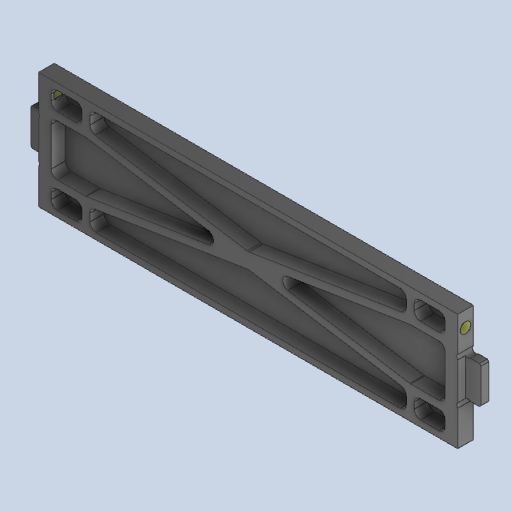
# Autodesk Inventor part: Cockpit_battery_frame
Saved by Autodesk Inventor 2022.3 (Build 263350000, 350)
## iProperties
Part Number: Cockpit_battery_frame
Material: アセタール樹脂、黒
Document SubType Name: Modeling
Designer: Masato Kubotera
Density: 1.425 g/cm^3
Appearance: 滑らか - 黒
Description: POM T5
Mass: 13.79 g
Surface Area: 149.623 cm^2
Volume: 9.6772 cm^3
Author: Masato Kubotera
Autodesk Inventor part; units mm, degrees
ref_plane "XZ Plane" through (0, 0, 0) normal (0, 1, 0) x (-1, 0, 0)
derived "Cockpit_side_frame.ipt"
sketch "スケッチ2" plane through (0, 0, 0) normal (0, 1, 0) x (-1, 0, 0)
  line L0 (-23.5, -22.5) -> (-28.5, -27.5)
  line L1 (-28.5, -27.5) -> (-28.5, -91)
  line L2 (-28.5, -91) -> (-23.5, -96)
  line L3 (-23.5, -96) -> (34.25, -96)
  line L4 (36.25, -98) -> (36.25, -128.5)
  line L5 (36.25, -128.5) -> (46.25, -138.5)
  line L6 (46.25, -138.5) -> (86.5, -138.5)
  line L7 (91.5, -133.5) -> (91.5, -20)
  line L8 (91.5, -20) -> (89, -17.5)
  line L9 (89, -17.5) -> (83.25, -17.5)
  line L10 (83.25, -17.5) -> (83.25, -21.0151)
  line L11 (81.7651, -22.5) -> (76.8599, -22.5)
  line L12 (75.375, -21.0151) -> (75.375, -17.5)
  line L13 (75.375, -17.5) -> (60.375, -17.5)
  line L14 (60.375, -17.5) -> (60.375, -21.0151)
  line L15 (58.8901, -22.5) -> (-23.5, -22.5)
  line L16 (-25.25, -25) -> (-20.25, -25) construction
  line L17 (-20.25, -25) -> (-20.25, -93.5) construction
  line L18 (-20.25, -93.5) -> (-25.25, -93.5) construction
  line L19 (-25.25, -93.5) -> (-25.25, -25) construction
  line L20 (-26, -25) -> (-25.25, -25) construction
  line L21 (-25.25, -93.5) -> (-26, -93.5) construction
  line L22 (-26, -93.5) -> (-26, -25) construction
  line L23 (-20.25, -93.5) -> (83.25, -93.5) construction
  line L24 (-20.25, -88.5) -> (83.25, -88.5) construction
  line L25 (83.25, -22.5) -> (83.25, -90) construction
  line L26 (83.25, -90) -> (88.25, -90) construction
  line L27 (88.25, -90) -> (88.25, -22.5) construction
  line L28 (83.25, -88.5) -> (83.25, -93.5) construction
  line L29 (83.25, -91) -> (88.25, -91) construction
  line L30 (88.25, -91) -> (88.25, -136) construction
  line L31 (83.25, -91) -> (83.25, -136) construction
  line L32 (83.25, -136) -> (88.25, -136) construction
  line L33 (38.75, -131) -> (38.75, -93.5) construction
  line L34 (43.75, -93.5) -> (43.75, -131) construction
  line L35 (38.75, -131) -> (43.75, -131) construction
  line L36 (41.25, -131) -> (41.25, -93.5) construction
  line L37 (43.75, -131) -> (81.25, -131) construction
  line L38 (81.25, -131) -> (81.25, -136) construction
  line L39 (81.25, -136) -> (43.75, -136) construction
  line L40 (43.75, -133.5) -> (81.25, -133.5) construction
  line L41 (85.75, -91) -> (85.75, -136) construction
  circle A0 centre (85.75, -133.5) radius 2.975
  arc A1 (83.25, -131) -> (88.25, -131) centre (85.75, -133.5) ccw construction
  line L42 (83.25, -91) -> (-20.25, -91) construction
  line L43 (41.25, -112.25) -> (43.75, -112.25) construction
  line L44 (62.5, -131) -> (62.5, -133.5) construction
  line L45 (41.2, -116.8151) -> (41.2, -107.6849)
  line L46 (43.8, -108.3) -> (43.8, -116.2)
  line L47 (43.8, -118.3) -> (41.2, -106.2) construction
  line L48 (41.2, -118.3) -> (43.8, -106.2) construction
  line L49 (58.55, -130.95) -> (66.45, -130.95)
  line L50 (67.0651, -133.55) -> (57.9349, -133.55)
  line L51 (56.45, -130.95) -> (68.55, -133.55) construction
  line L52 (68.55, -130.95) -> (56.45, -133.55) construction
  line L53 (41.25, -106.25) -> (43.75, -106.25) construction
  line L54 (41.25, -118.25) -> (43.75, -118.25) construction
  arc A2 (42.6849, -106.2) -> (41.2, -107.6849) centre (41.9425, -106.9425) ccw
  arc A3 (43.8, -108.3) -> (43.8, -106.2) centre (43.8, -107.25) ccw
  arc A4 (41.2, -116.8151) -> (42.6849, -118.3) centre (41.9425, -117.5575) ccw
  arc A5 (43.8, -118.3) -> (43.8, -116.2) centre (43.8, -117.25) ccw
  line L55 (56.5, -133.5) -> (56.5, -131) construction
  line L56 (68.5, -131) -> (68.5, -133.5) construction
  arc A6 (56.45, -132.0651) -> (57.9349, -133.55) centre (57.1925, -132.8075) ccw
  arc A7 (58.55, -130.95) -> (56.45, -130.95) centre (57.5, -130.95) ccw
  arc A8 (67.0651, -133.55) -> (68.55, -132.0651) centre (67.8075, -132.8075) ccw
  arc A9 (68.55, -130.95) -> (66.45, -130.95) centre (67.5, -130.95) ccw
  line L57 (56.45, -132.0651) -> (56.45, -130.95)
  line L58 (68.55, -130.95) -> (68.55, -132.0651)
  line L59 (42.6849, -106.2) -> (43.8, -106.2)
  line L60 (43.8, -118.3) -> (42.6849, -118.3)
  circle A10 centre (48.75, -133.5) radius 1.6
  line L61 (88.25, -22.5) -> (88.25, -17.5) construction
  line L62 (89, -17.5) -> (89, -90) construction
  line L63 (89, -90) -> (88.25, -90) construction
  line L64 (-13.5, -82.5) -> (-13.5, -61)
  arc A11 (-13.5, -82.5) -> (-11.5, -84.5) centre (-11.5, -82.5) ccw
  line L65 (45.5, -84.5) -> (-11.5, -84.5)
  arc A12 (45.5, -84.5) -> (47.5, -82.5) centre (45.5, -82.5) ccw
  line L66 (47.5, -61) -> (47.5, -82.5)
  arc A13 (47.5, -61) -> (45.5, -59) centre (45.5, -61) ccw
  line L67 (-11.5, -59) -> (45.5, -59)
  arc A14 (-11.5, -59) -> (-13.5, -61) centre (-11.5, -61) ccw
  line L68 (31.5, -88.5) -> (31.5, -91) construction
  line L69 (85.75, -22.5) -> (85.75, -90) construction
  circle A15 centre (85.75, -31.25) radius 1.6
  circle A16 centre (85.75, -31.25) radius 3
  circle A17 centre (85.75, -81.25) radius 3
  circle A18 centre (85.75, -81.25) radius 1.6
  line L70 (88.25, -22.5) -> (83.25, -22.5) construction
  arc A19 (88.25, -91) -> (83.25, -91) centre (85.75, -133.5) ccw construction
  circle A20 centre (48.75, -133.5) radius 3
  circle A21 centre (41.25, -98.5) radius 1.6
  circle A22 centre (41.25, -98.5) radius 3
  line L71 (10.55, -88.5) -> (10.55, -91) construction
  line L72 (52.45, -88.5) -> (52.45, -91) construction
  line L73 (51.0151, -91.05) -> (11.9849, -91.05)
  line L74 (10.5, -89.5651) -> (10.5, -88.45)
  line L75 (12.6, -88.45) -> (50.4, -88.45)
  line L76 (52.5, -88.45) -> (52.5, -89.5651)
  line L77 (52.5, -91.05) -> (10.5, -88.45) construction
  line L78 (10.5, -91.05) -> (52.5, -88.45) construction
  arc A23 (12.6, -88.45) -> (10.5, -88.45) centre (11.55, -88.45) ccw
  arc A24 (10.5, -89.5651) -> (11.9849, -91.05) centre (11.2425, -90.3075) ccw
  arc A25 (51.0151, -91.05) -> (52.5, -89.5651) centre (51.7575, -90.3075) ccw
  arc A26 (52.5, -88.45) -> (50.4, -88.45) centre (51.45, -88.45) ccw
  line L79 (-20.25, -31) -> (83.25, -31) construction
  line L80 (83.25, -26) -> (-20.25, -26) construction
  line L81 (-20.25, -26) -> (-20.25, -31) construction
  line L82 (-20.25, -28.5) -> (83.25, -28.5) construction
  line L83 (31.5, -31) -> (31.5, -26) construction
  line L84 (11.9849, -31) -> (51.0151, -31)
  arc A27 (10.5, -29.5151) -> (11.9849, -31) centre (11.2425, -30.2575) ccw
  arc A28 (51.0151, -31) -> (52.5, -29.5151) centre (51.7575, -30.2575) ccw
  line L85 (10.55, -31) -> (10.55, -26) construction
  line L86 (52.45, -26) -> (52.45, -31) construction
  circle A29 centre (6.5, -28.5) radius 1.6
  circle A30 centre (6.5, -28.5) radius 3
  line L87 (-26, -59.25) -> (-25.25, -59.25) construction
  line L88 (-22.75, -25) -> (-22.75, -93.5) construction
  arc A31 (58.8901, -22.5) -> (60.375, -21.0151) centre (59.6325, -21.7575) ccw
  arc A32 (75.375, -21.0151) -> (76.8599, -22.5) centre (76.1175, -21.7575) ccw
  line L89 (56.4375, -22.5) -> (56.4375, -17.5) construction
  line L90 (79.3125, -22.5) -> (79.3125, -17.5) construction
  circle A33 centre (-22.75, -31.75) radius 1.6
  circle A34 centre (-22.75, -31.75) radius 3
  circle A35 centre (-22.75, -86.75) radius 1.6
  circle A36 centre (-22.75, -86.75) radius 3
  line L91 (60.375, -22.5) -> (75.375, -22.5)
  line L92 (52.5, -17.5) -> (52.5, -22.5) construction
  circle A37 centre (85.75, -98.5) radius 1.475
  circle A38 centre (85.75, -103.5) radius 1.475
  circle A39 centre (85.75, -108.5) radius 1.475
  line L93 (59.5, -88.5) -> (78.75, -88.5)
  line L94 (80.75, -90.5) -> (80.75, -126.5)
  line L95 (78.75, -128.5) -> (48.25, -128.5)
  line L96 (46.25, -126.5) -> (46.25, -110)
  arc A40 (46.25, -126.5) -> (48.25, -128.5) centre (48.25, -126.5) ccw
  arc A41 (78.75, -128.5) -> (80.75, -126.5) centre (78.75, -126.5) ccw
  arc A42 (80.75, -90.5) -> (78.75, -88.5) centre (78.75, -90.5) ccw
  arc A43 (36.25, -98) -> (34.25, -96) centre (34.25, -98) ccw
  circle A44 centre (-13.5, -55) radius 1.75
  circle A45 centre (-13.5, -55) radius 2
  line L97 (23.9, -43.85) -> (10.1, -43.85) construction
  line L98 (10.1, -43.85) -> (10.1, -34.65) construction
  line L99 (10.1, -34.65) -> (23.9, -34.65) construction
  line L100 (23.9, -34.65) -> (23.9, -43.85) construction
  line L101 (23.9, -43.85) -> (10.1, -34.65) construction
  line L102 (10.1, -43.85) -> (23.9, -34.65) construction
  line L103 (9.45, -33.95) -> (24.55, -33.95) construction
  line L104 (24.55, -33.95) -> (24.55, -44.55) construction
  line L105 (24.55, -44.55) -> (9.45, -44.55) construction
  line L106 (9.45, -44.55) -> (9.45, -33.95) construction
  line L107 (9.45, -33.95) -> (24.55, -44.55) construction
  line L108 (24.55, -33.95) -> (9.45, -44.55) construction
  line L109 (10.8849, -33.9) -> (23.1151, -33.9)
  line L110 (24.6, -35.3849) -> (24.6, -43.1151)
  line L111 (24.6, -44.6) -> (9.4, -33.9) construction
  line L112 (9.4, -44.6) -> (24.6, -33.9) construction
  line L113 (23.95, -43.9) -> (10.05, -34.6) construction
  line L114 (10.05, -43.9) -> (23.95, -34.6) construction
  arc A46 (10.8849, -33.9) -> (9.4, -35.3849) centre (10.1425, -34.6425) ccw
  arc A47 (11.5349, -34.6) -> (10.05, -36.0849) centre (10.7925, -35.3425) ccw
  line L115 (9.4, -39.25) -> (24.6, -39.25) construction
  line L116 (17, -33.9) -> (17, -44.6) construction
  arc A48 (24.6, -35.3849) -> (23.1151, -33.9) centre (23.8575, -34.6425) ccw
  arc A49 (23.95, -36.0849) -> (22.4651, -34.6) centre (23.2075, -35.3425) ccw
  arc A50 (10.05, -42.4151) -> (11.5349, -43.9) centre (10.7925, -43.1575) ccw
  arc A51 (9.4, -43.1151) -> (10.8849, -44.6) centre (10.1425, -43.8575) ccw
  arc A52 (22.4651, -43.9) -> (23.95, -42.4151) centre (23.2075, -43.1575) ccw
  arc A53 (23.1151, -44.6) -> (24.6, -43.1151) centre (23.8575, -43.8575) ccw
  line L117 (11.5349, -34.6) -> (22.4651, -34.6)
  line L118 (23.95, -36.0849) -> (23.95, -42.4151)
  line L119 (9.4, -43.1151) -> (9.4, -35.3849)
  line L120 (10.05, -42.4151) -> (10.05, -36.0849)
  line L121 (22.4651, -43.9) -> (11.5349, -43.9)
  line L122 (23.1151, -44.6) -> (10.8849, -44.6)
  line L123 (-13.5, -71.75) -> (47.5, -71.75) construction
  line L124 (85.75, -56.25) -> (88.25, -56.25) construction
  line L125 (85.7, -69.2) -> (85.7, -43.3)
  line L126 (88.3049, -71.3569) -> (85.7, -41.2) construction
  line L127 (85.7, -71.3) -> (88.3, -41.2) construction
  arc A54 (85.7, -41.2) -> (85.7, -43.3) centre (85.7, -42.25) ccw
  arc A55 (88.3, -42.6849) -> (86.8151, -41.2) centre (87.5575, -41.9425) ccw
  arc A56 (85.7, -69.2) -> (85.7, -71.3) centre (85.7, -70.25) ccw
  arc A57 (86.8151, -71.3) -> (88.3, -69.8151) centre (87.5575, -70.5575) ccw
  line L128 (85.75, -41.25) -> (88.25, -41.25) construction
  line L129 (85.75, -71.25) -> (88.25, -71.25) construction
  line L130 (88.3, -42.6849) -> (88.3, -69.8151)
  line L131 (88.3, -66.8652) -> (88.3, -69.8151)
  line L132 (86.8151, -71.3) -> (85.7, -71.3)
  line L133 (85.7, -41.2) -> (86.8151, -41.2)
  line L134 (86.5, -138.5) -> (91.5, -133.5)
  arc A58 (81.7651, -22.5) -> (83.25, -21.0151) centre (82.5075, -21.7575) ccw
  circle A59 centre (85.75, -93.5) radius 2
  circle A60 centre (85.75, -93.5) radius 4 construction
  arc A61 (-13.5, -49) -> (-11.5, -51) centre (-11.5, -49) ccw construction
  line L135 (45.5, -51) -> (-11.5, -51) construction
  arc A62 (45.5, -51) -> (47.5, -49) centre (45.5, -49) ccw construction
  line L136 (10.5, -29.5151) -> (10.5, -22.5)
  line L137 (52.5, -29.5151) -> (52.5, -22.5)
  line L138 (67.875, -17.5) -> (67.875, -22.5) construction
  line L139 (52.5, -17.5) -> (83.25, -17.5) construction
  line L140 (43.75, -131) -> (43.75, -136) construction
  line L141 (57.5, -22.5) -> (57.5, -103) construction
  line L142 (57.5, -103) -> (52.5, -108) construction
  line L143 (-23.5, -108) -> (52.5, -108) construction
  line L144 (57.5, -90.5) -> (57.5, -103)
  line L145 (57.5, -103) -> (52.5, -108)
  line L146 (52.5, -108) -> (48.25, -108)
  arc A63 (59.5, -88.5) -> (57.5, -90.5) centre (59.5, -90.5) ccw
  arc A64 (48.25, -108) -> (46.25, -110) centre (48.25, -110) ccw
  circle A65 centre (56.5, -28.5) radius 3
  circle A66 centre (56.5, -28.5) radius 1.6
  line L147 (-13.5, -49) -> (-13.5, -29.5)
  point P0 (0, 0)
  point P1 (-25.7227, -96)
  point P2 (-23.5, -22.5)
  point P3 (42.5, -112.25)
  point P4 (62.5, -132.25)
  point P5 (31.5, -89.75)
  point P6 (31.5, -28.5)
  point P7 (52.5, -22)
  point P8 (46.25, -108)
  point P9 (57.5, -88.5)
  point P10 (17, -39.25)
  point P11 (17, -39.25)
  point P12 (87, -56.25)
  point P13 (17, -51)
  point P14 (10.5, -31)
  point P15 (-13.5, -39.25)
  dimension "d1" = 43.75
  dimension "d2" = 5
  dimension "d3" = 2.5
  measures "d1" distance from line of point (0, 0) L34
  measures "d2" distance of L34.end L33.start
  measures "d3" distance of L54.start L54.end
ref_plane "作業平面1" through (-43.75, 0, 0) normal (1, 0, 0) x (0, 1, 0)
sketch "スケッチ3" plane through (-43.75, 0, 0) normal (1, 0, 0) x (0, 1, 0)
  line L0 (-135, -93.5) -> (0, -93.5)
  line L1 (0, -131) -> (-135, -131)
  line L2 (1.4849, -106.25) -> (5, -106.25)
  line L3 (5, -106.25) -> (5, -118.25)
  arc A0 (0, -104.7651) -> (1.4849, -106.25) centre (0.7425, -105.5075) ccw
  line L4 (0, -93.5) -> (0, -104.7651)
  line L5 (-134.9908, -112.25) -> (0, -112.25) construction
  line L6 (1.4849, -118.25) -> (5, -118.25)
  arc A1 (1.4849, -118.25) -> (0, -119.7349) centre (0.7425, -118.9925) ccw
  line L7 (0, -131) -> (0, -119.7349)
  line L8 (0, -106.25) -> (0, -118.25)
  line L9 (0, -119.7349) -> (0, -131)
  line L10 (-67.5, -93.5) -> (-67.5, -131) construction
  line L11 (-136.4849, -106.25) -> (-140, -106.25)
  line L12 (-140, -106.25) -> (-140, -118.25)
  arc A2 (-136.4849, -106.25) -> (-135, -104.7651) centre (-135.7425, -105.5075) ccw
  line L13 (-135, -93.5) -> (-135, -104.7651)
  line L14 (-136.4849, -118.25) -> (-140, -118.25)
  arc A3 (-135, -119.7349) -> (-136.4849, -118.25) centre (-135.7425, -118.9925) ccw
  line L15 (-135, -131) -> (-135, -119.7349)
  line L16 (-135, -106.25) -> (-135, -118.25)
  line L17 (-135, -119.7349) -> (-135, -131)
  line L18 (-12, -123) -> (-6, -123)
  line L19 (-4, -125) -> (-4, -127)
  line L20 (-6, -129) -> (-12, -129)
  line L21 (-14, -127) -> (-14, -125)
  line L22 (-4, -118.5) -> (-4, -106)
  line L23 (-67.186, -114.7748) -> (-18.186, -122.5646)
  line L24 (-16.5, -124.5398) -> (-16.5, -127)
  line L25 (-18.5, -129) -> (-116.5, -129)
  line L26 (-6, -120.5) -> (-15.092, -120.5)
  line L27 (-15.406, -120.4752) -> (-54.7201, -114.2252)
  line L28 (-12, -101.5) -> (-6, -101.5)
  line L29 (-4, -99.5) -> (-4, -97.5)
  line L30 (-6, -95.5) -> (-12, -95.5)
  line L31 (-14, -97.5) -> (-14, -99.5)
  line L32 (-67.186, -109.7252) -> (-18.186, -101.9354)
  line L33 (-16.5, -99.9602) -> (-16.5, -97.5)
  line L34 (-18.5, -95.5) -> (-116.5, -95.5)
  line L35 (-6, -104) -> (-15.092, -104)
  line L36 (-15.406, -104.0248) -> (-54.7201, -110.2748)
  line L37 (-67.814, -114.7748) -> (-116.814, -122.5646)
  line L38 (-118.5, -124.5398) -> (-118.5, -127)
  line L39 (-118.5, -99.9602) -> (-118.5, -97.5)
  line L40 (-67.814, -109.7252) -> (-116.814, -101.9354)
  arc A4 (-6, -129) -> (-4, -127) centre (-6, -127) ccw
  arc A5 (-4, -125) -> (-6, -123) centre (-6, -125) ccw
  arc A6 (-12, -123) -> (-14, -125) centre (-12, -125) ccw
  arc A7 (-14, -127) -> (-12, -129) centre (-12, -127) ccw
  arc A8 (-18.5, -129) -> (-16.5, -127) centre (-18.5, -127) ccw
  arc A9 (-16.5, -124.5398) -> (-18.186, -122.5646) centre (-18.5, -124.5398) ccw
  arc A10 (-67.186, -114.7748) -> (-67.814, -114.7748) centre (-67.5, -116.75) ccw
  arc A11 (-116.814, -122.5646) -> (-118.5, -124.5398) centre (-116.5, -124.5398) ccw
  arc A12 (-118.5, -127) -> (-116.5, -129) centre (-116.5, -127) ccw
  arc A13 (-118.5, -99.9602) -> (-116.814, -101.9354) centre (-116.5, -99.9602) ccw
  arc A14 (-116.5, -95.5) -> (-118.5, -97.5) centre (-116.5, -97.5) ccw
  arc A15 (-16.5, -97.5) -> (-18.5, -95.5) centre (-18.5, -97.5) ccw
  arc A16 (-18.186, -101.9354) -> (-16.5, -99.9602) centre (-18.5, -99.9602) ccw
  arc A17 (-67.814, -109.7252) -> (-67.186, -109.7252) centre (-67.5, -107.75) ccw
  arc A18 (-54.7201, -110.2748) -> (-54.7201, -114.2252) centre (-54.4061, -112.25) ccw
  arc A19 (-15.092, -104) -> (-15.406, -104.0248) centre (-15.092, -106) ccw
  arc A20 (-4, -106) -> (-6, -104) centre (-6, -106) ccw
  arc A21 (-6, -120.5) -> (-4, -118.5) centre (-6, -118.5) ccw
  arc A22 (-15.406, -120.4752) -> (-15.092, -120.5) centre (-15.092, -118.5) ccw
  arc A23 (-14, -99.5) -> (-12, -101.5) centre (-12, -99.5) ccw
  arc A24 (-12, -95.5) -> (-14, -97.5) centre (-12, -97.5) ccw
  arc A25 (-4, -97.5) -> (-6, -95.5) centre (-6, -97.5) ccw
  arc A26 (-6, -101.5) -> (-4, -99.5) centre (-6, -99.5) ccw
  line L41 (-123, -123) -> (-129, -123)
  line L42 (-121, -127) -> (-121, -125)
  line L43 (-131, -118.5) -> (-131, -106)
  line L44 (-129, -120.5) -> (-119.908, -120.5)
  line L45 (-119.594, -120.4752) -> (-80.2799, -114.2252)
  line L46 (-123, -101.5) -> (-129, -101.5)
  line L47 (-121, -97.5) -> (-121, -99.5)
  line L48 (-129, -95.5) -> (-123, -95.5)
  line L49 (-131, -99.5) -> (-131, -97.5)
  line L50 (-119.594, -104.0248) -> (-80.2799, -110.2748)
  line L51 (-129, -104) -> (-119.908, -104)
  arc A27 (-131, -127) -> (-129, -129) centre (-129, -127) ccw
  arc A28 (-129, -123) -> (-131, -125) centre (-129, -125) ccw
  arc A29 (-121, -125) -> (-123, -123) centre (-123, -125) ccw
  arc A30 (-123, -129) -> (-121, -127) centre (-123, -127) ccw
  arc A31 (-80.2799, -114.2252) -> (-80.2799, -110.2748) centre (-80.5939, -112.25) ccw
  arc A32 (-119.594, -104.0248) -> (-119.908, -104) centre (-119.908, -106) ccw
  arc A33 (-129, -104) -> (-131, -106) centre (-129, -106) ccw
  arc A34 (-131, -118.5) -> (-129, -120.5) centre (-129, -118.5) ccw
  arc A35 (-119.908, -120.5) -> (-119.594, -120.4752) centre (-119.908, -118.5) ccw
  arc A36 (-123, -101.5) -> (-121, -99.5) centre (-123, -99.5) ccw
  arc A37 (-121, -97.5) -> (-123, -95.5) centre (-123, -97.5) ccw
  arc A38 (-129, -95.5) -> (-131, -97.5) centre (-129, -97.5) ccw
  arc A39 (-131, -99.5) -> (-129, -101.5) centre (-129, -99.5) ccw
  line L52 (-129, -129) -> (-123, -129)
  line L53 (-4, -98.5) -> (0, -98.5) construction
  line L54 (-131, -125) -> (-131, -127)
  point P0 (0, 0)
  point P1 (-135, -112.25)
  point P2 (-14, -123)
  point P3 (-4, -129)
  point P4 (-4, -123)
  point P5 (-14, -129)
  point P6 (-4, -120.5)
  point P7 (-67.5, -114.7249)
  point P8 (-16.5, -122.8327)
  point P9 (-16.5, -129)
  point P10 (-118.5, -129)
  point P11 (-15.25, -120.5)
  point P12 (-67.1445, -112.25)
  point P13 (-14, -101.5)
  point P14 (-4, -95.5)
  point P15 (-4, -101.5)
  point P16 (-14, -95.5)
  point P17 (-4, -104)
  point P18 (-67.5, -109.7751)
  point P19 (-16.5, -101.6673)
  point P20 (-16.5, -95.5)
  point P21 (-15.25, -104)
  point P22 (-118.5, -122.8327)
  point P23 (-118.5, -129)
  point P24 (-118.5, -101.6673)
  point P25 (-118.5, -95.5)
  dimension "d5" = 5
  dimension "d6" = 135
  dimension "d7" = 1.05
  dimension "d19" = 4
  dimension "d20" = 2
  dimension "d21" = 10
  dimension "d22" = 2.5
  dimension "d23" = 11.25
  dimension "d24" = 2.5
  dimension "d25" = 2
  dimension "d26" = 2.5
  dimension "d27" = 5
  constraints: 110 end point, 85 point on circle, 72 symmetric about line, 58 point on line, 46 tangent, 40 centre point, 22 equal radius, 9 perpendicular, 5 midpoint, 5 parallel, 4 horizontal, 3 coincident, 2 collinear, 1 vertical, 16 other
  measures "d5" distance between parallel lines of L3 L8
  measures "d6" distance of L0.start L0.end
  measures "d7" radius of A0
  measures "d19" distance between parallel lines of L7 L19
  measures "d20" distance between parallel lines of L1 L20
  measures "d21" distance of point (-4, -129) point (-14, -129)
  measures "d22" distance between parallel lines of L24 L21
  measures "d23" distance of point (-4, -120.5) point (-15.25, -120.5)
  measures "d24" distance between parallel lines of L23 L27
  measures "d25" radius of A4
  measures "d26" distance between parallel lines of L18 L26
extrude "押し出し1" add sketch "スケッチ3" along normal blind 5 contours L0 L4 A0 L8 A1 L7 L1 L15 A3 L16 A2 L13
extrude "押し出し2" add sketch "スケッチ3" along normal blind 2.5 contours L16 A3 L14 L12 L11 A2 | A0 L2 L3 L6 A1 L8
hole "穴1" at (-41.25, 0, -98.5) direction (0, -1, 0) diameter 3.4587 depth 4 thread size "M4x0.5" class "6H" standard "ANSI Metric M Profile"
ref_plane "作業平面2" through (-43.75, -67.5, -93.5) normal (0, 1, 0) x (1, 0, 0)
mirror "ミラー1" about plane through (-43.75, -67.5, -93.5) normal (0, 1, 0) of "穴1"
extrude "押し出し3" add sketch "スケッチ3" along normal blind 0.5 contours L18 A5 L19 A4 L20 A7 L21 A6 | A21 L26 A22 L27 A18 L36 A19 L35 A20 L22 | L23 A9 L24 A8 L25 A12 L38 A11 L37 A10 | A23 L31 A24 L30 A25 L29 A26 L28 | A17 L40 A13 L39 A14 L34 A15 L33 A16 L32 | A29 L42 A30 L52 A27 L54 A28 L41 | L43 A33 L51 A32 L50 A31 L45 A35 L44 A34 | L46 A39 L49 A38 L48 A37 L47 A36
chamfer "面取り1" distance 0.5 angle 45 4 edges at (-42.5, -140, -118.25) (-42.5, -140, -106.25) (-42.5, 5, -118.25) (-42.5, 5, -106.25)
equation "\"d23\" = d21 + 0.5 * d22"
equation "\"d24\" = d22"
equation "\"d26\" = d22"
equation "\"d27\" = 2 * d22"
equation "\"d8\" = d2"
equation "\"d10\" = d3"
equation "\"d4\" = -d1"
